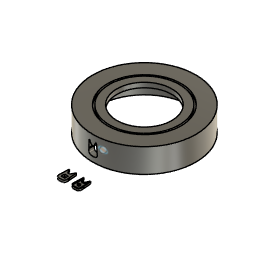
PLAtaforma v2 (Autodesk Fusion 360 design; units mm, degrees)
Autodesk Fusion 360 part; units mm, degrees
sketch "Boceto1" plane through (0, 0, 0) normal (0, 0, 1) x (1, 0, 0)
  circle A0 centre (-125, 125) radius 55.5
sketch "Boceto2" plane through (0, 0, 0) normal (0, 0, 1) x (1, 0, 0)
  circle A0 centre (0, 27.0396) radius 57.4187
  circle A1 centre (150, 200) radius 57.5
extrude "Extruir3" add sketch "Boceto2" along normal blind 35 contours A1 makes body 1
move_body "Desplazar4" bodies 1 to x (1, 0, 0) y (0, 1, 0) z (0, 0, 1) at (-150, -175, 50)
sketch "Boceto3" plane through (0, 0, 85) normal (0, 0, 1) x (-1, 0, 0)
  circle A0 centre (0, -25) radius 57.5
  circle A1 centre (0, -25) radius 40
  constraint concentric A0 A1
extrude "Extruir4" cut sketch "Boceto3" against normal blind 40 contours A1 bodies 1
sketch "Boceto4" plane through (0, 0, 85) normal (0, 0, 1) x (-1, 0, 0)
  circle A0 centre (0, -25) radius 40
  circle A1 centre (0, -25) radius 57.5
move_body "Desplazar5" bodies 1 to x (1, 0, 0) y (0, 1, 0) z (0, 0, 1) at (0, 0, -140)
sketch "Boceto5" plane through (0, 0, -55) normal (0, 0, 1) x (-1, 0, 0)
  circle A0 centre (0, -25) radius 40
  circle A1 centre (0, -25) radius 57.5
  circle A2 centre (0, -25) radius 53.4509
  circle A3 centre (0, -25) radius 51
  constraint concentric A0 A2
  constraint concentric A0 A3
extrude "Extruir5" cut sketch "Boceto5" against normal blind 3 contours A2 bodies 1
fillet "Empalme1" radius 0.25 1 edges at (49.8337, 5.6713, -58) on bodies 1
fillet "Empalme2" radius 0.25 1 edges at (47.5487, 43.4424, -58) on bodies 1
sketch "Boceto6" plane through (0, 0, -55) normal (0, 0, 1) x (-1, 0, 0)
  circle A0 centre (0, -25) radius 51
  circle A1 centre (0, -25) radius 40
  line L0 (100, -175) -> (45.9317, -175)
  line L1 (45.9317, -175) -> (45.9317, -137.795)
  line L2 (45.9317, -137.795) -> (100, -137.795)
  line L3 (100, -137.795) -> (100, -175)
  constraint horizontal L0
  constraint vertical L1
  constraint horizontal L2
  constraint vertical L3
sketch "Boceto7" plane through (0, 0, 0) normal (0, 1, 0) x (1, 0, 0)
  spline S0 degree 5 poles (-6, -14) (-6.016, -13.81) (-6.046, -13.4349) (-6.0844, -12.8873) (-6.1226, -12.187) (-6.143, -11.3625) (-6.116, -10.5901) (-6.0091, -9.873) (-5.7505, -9.2135) (-5.2931, -8.6238) (-4.6335, -8.1243) (-3.7909, -7.7338) (-2.8029, -7.4645) (-1.7133, -7.3125) (-0.5683, -7.2594) (0.5856, -7.2827) (1.7041, -7.3621) (2.7474, -7.489) (3.6824, -7.6725) (4.4854, -7.9512) (5.1429, -8.3847) (5.6471, -9.0113) (5.9972, -9.8345) (6.1897, -10.7563) (6.235, -11.6318) (6.1815, -12.4467) (6.1039, -13.0649) (6.0484, -13.5294) (6.0154, -13.8425) (6, -14) knots 0 0 0 0 0 0 0.04 0.08 0.12 0.16 0.2 0.24 0.28 0.32 0.36 0.4 0.44 0.48 0.52 0.56 0.6 0.64 0.68 0.72 0.76 0.8 0.84 0.88 0.92 0.96 1 1 1 1 1 1
  line L0 (6.1425, -12.5468) -> (5.8575, -15.4532)
  line L1 (5.5566, -8.4249) -> (6.4434, -11.5751)
  line L2 (-6.2996, -11.2694) -> (-5.7004, -8.7306)
  spline S1 degree 5 poles (-5.8636, -15.4223) (-5.8656, -16.3931) (-5.8678, -18.2327) (-5.8657, -20.6855) (-5.8432, -23.3299) (-5.7393, -25.5443) (-5.5105, -26.6441) (-5.1266, -26.6944) (-4.5821, -25.8579) (-3.9459, -24.5382) (-3.2994, -23.1771) (-2.6763, -22.0178) (-2.1679, -21.2779) (-1.777, -20.8414) (-1.5201, -20.6109) (-1.4081, -20.5209) knots 0 0 0 0 0 0 0.04 0.08 0.12 0.16 0.2 0.24 0.28 0.32 0.36 0.4 0.430271 0.430271 0.430271 0.430271 0.430271 0.430271
  line L3 (-5.8558, -11.6968) -> (-5.8714, -19.1478)
  line L4 (-4.7611, -26.105) -> (-4.2835, -25.2366)
  ellipse E0 centre (0, -14) end of major axis (6, -14) minor radius 6.7082 (-6, -14) -> (-5.8636, -15.4223) ccw
  ellipse E1 centre (0, -14) end of major axis (6, -14) minor radius 6.7082 (-1.4081, -20.5209) -> (1.0288, -20.6089) ccw
  ellipse E2 centre (0, -14) end of major axis (6, -14) minor radius 6.7082 (5.8575, -15.4532) -> (6, -14) ccw
  spline S2 degree 5 poles (1.0288, -20.6089) (1.0454, -20.6251) (1.2133, -20.7918) (1.5263, -21.1625) (1.9673, -21.8512) (2.5023, -22.9747) (3.0752, -24.4534) (3.5768, -25.7819) (4.0187, -26.6987) (4.4124, -26.9878) (4.766, -26.5076) (5.0852, -25.1698) (5.3736, -22.9285) (5.5812, -20.3988) (5.7243, -18.0869) (5.814, -16.3617) (5.8575, -15.4532) knots 0.555614 0.555614 0.555614 0.555614 0.555614 0.555614 0.56 0.6 0.64 0.68 0.72 0.76 0.8 0.84 0.88 0.92 0.96 1 1 1 1 1 1
  line L5 (0.2621, -19.8617) -> (1.7954, -21.356)
  line L6 (5.6884, -18.9867) -> (6.0267, -11.9197)
  spline S3 degree 3 poles (-1.4604, -20.264) (-0.626, -20.5082) (0.2565, -20.5396) (1.1028, -20.3557) knots 2.884408 2.884408 2.884408 2.884408 3.334897 3.334897 3.334897 3.334897
  spline S4 degree 3 poles (1.1028, -20.3557) (1.1323, -20.3844) (1.1619, -20.4132) (1.1914, -20.442) (1.9144, -21.1466) (2.5155, -22.4275) (3.0242, -23.696) (3.3295, -24.4573) (3.6018, -25.1998) (3.8432, -25.7413) (4.0212, -26.1408) (4.1959, -26.4325) (4.2994, -26.53) (4.3198, -26.5492) (4.3362, -26.5607) (4.346, -26.5662) knots 0.550938 0.550938 0.550938 0.550938 0.555614 0.555614 0.555614 0.661996 0.661996 0.661996 0.725847 0.725847 0.725847 0.772953 0.772953 0.772953 0.78222 0.78222 0.78222 0.78222
  spline S5 degree 3 poles (4.346, -26.5662) (4.3827, -26.5368) (4.4823, -26.3889) (4.5725, -26.1162) (4.9775, -24.8912) (5.343, -21.3299) (5.6248, -15.4421) (5.6251, -15.4363) (5.6253, -15.4305) (5.6256, -15.4247) knots 0.80969 0.80969 0.80969 0.80969 0.844339 0.844339 0.844339 1 1 1 1.000153 1.000153 1.000153 1.000153
  spline S6 degree 3 poles (5.6256, -15.4247) (5.7202, -14.954) (5.7677, -14.4713) (5.767, -13.9887) knots -1.791812 -1.791812 -1.791812 -1.791812 -1.569057 -1.569057 -1.569057 -1.569057
  spline S7 degree 3 poles (-5.767, -13.9903) (-5.7673, -13.987) (-5.7676, -13.9837) (-5.7678, -13.9804) (-5.8747, -12.715) (-5.9561, -11.5732) (-5.8629, -10.6164) (-5.7828, -9.7954) (-5.5171, -9.1267) (-4.8246, -8.5921) (-4.0701, -8.0096) (-2.8284, -7.6532) (-1.4477, -7.5498) (-0.0784, -7.4473) (1.4043, -7.5365) (2.616, -7.7229) (3.7061, -7.8906) (4.542, -8.1517) (5.0887, -8.7456) (5.479, -9.1697) (5.7466, -9.8087) (5.8761, -10.4922) (6.0308, -11.3093) (5.9793, -12.0858) (5.8969, -12.8241) (5.8544, -13.2054) (5.8064, -13.5869) (5.7681, -13.9773) (5.7677, -13.9811) (5.7674, -13.9849) (5.767, -13.9887) knots -0.000415 -0.000415 -0.000415 -0.000415 0 0 0 0.160546 0.160546 0.160546 0.298298 0.298298 0.298298 0.448379 0.448379 0.448379 0.597213 0.597213 0.597213 0.731122 0.731122 0.731122 0.82672 0.82672 0.82672 0.940992 0.940992 0.940992 1 1 1 1.000581 1.000581 1.000581 1.000581
  spline S8 degree 3 poles (-5.767, -13.9903) (-5.7676, -14.4639) (-5.7217, -14.9376) (-5.6305, -15.4) knots 1.569298 1.569298 1.569298 1.569298 1.787916 1.787916 1.787916 1.787916
  spline S9 degree 3 poles (-5.6305, -15.4) (-5.6306, -15.4076) (-5.6306, -15.4152) (-5.6306, -15.4228) (-5.6379, -18.9007) (-5.6384, -21.5996) (-5.58, -23.4507) (-5.5465, -24.5102) (-5.4905, -25.2917) (-5.4051, -25.7776) (-5.3556, -26.0591) (-5.2879, -26.2439) (-5.248, -26.3044) knots -0.000188 -0.000188 -0.000188 -0.000188 0 0 0 0.085991 0.085991 0.085991 0.13521 0.13521 0.13521 0.163732 0.163732 0.163732 0.163732
  spline S10 degree 3 poles (-5.248, -26.3044) (-5.1951, -26.267) (-5.0881, -26.1485) (-4.9745, -25.9761) (-4.6357, -25.4621) (-4.1975, -24.5076) (-3.7667, -23.6307) (-3.1866, -22.4499) (-2.5988, -21.3794) (-1.925, -20.6804) (-1.8044, -20.5553) (-1.6809, -20.4412) (-1.554, -20.3392) (-1.5228, -20.3142) (-1.4916, -20.2891) (-1.4604, -20.264) knots 0.197683 0.197683 0.197683 0.197683 0.224372 0.224372 0.224372 0.303955 0.303955 0.303955 0.411102 0.411102 0.411102 0.430271 0.430271 0.430271 0.435327 0.435327 0.435327 0.435327
  spline S11 degree 3 poles (-1.6069, -19.4391) (-0.6663, -19.7925) (0.3605, -19.8343) (1.3181, -19.5394) knots 2.809731 2.809731 2.809731 2.809731 3.412393 3.412393 3.412393 3.412393
  spline S12 degree 3 poles (1.3181, -19.5394) (1.4468, -19.6649) (1.5756, -19.7903) (1.7043, -19.9157) (2.5333, -20.7237) (3.1086, -21.9593) (3.6075, -23.1786) (3.8069, -23.6658) (3.9901, -24.1463) (4.1575, -24.5734) knots 0.535231 0.535231 0.535231 0.535231 0.555614 0.555614 0.555614 0.655325 0.655325 0.655325 0.695165 0.695165 0.695165 0.695165
  spline S13 degree 3 poles (4.1575, -24.5734) (4.3953, -23.0694) (4.6167, -20.5464) (4.8059, -17.071) (4.8349, -16.5389) (4.8632, -15.9842) (4.8908, -15.4069) (4.892, -15.3822) (4.8932, -15.3574) (4.8944, -15.3327) knots 0.884759 0.884759 0.884759 0.884759 0.984699 0.984699 0.984699 1 1 1 1.000654 1.000654 1.000654 1.000654
  spline S14 degree 3 poles (4.8944, -15.3327) (4.9887, -14.8822) (5.0352, -14.418) (5.032, -13.9543) knots -1.801106 -1.801106 -1.801106 -1.801106 -1.562974 -1.562974 -1.562974 -1.562974
  spline S15 degree 3 poles (-5.0321, -13.9606) (-5.0332, -13.9466) (-5.0344, -13.9326) (-5.0356, -13.9186) (-5.1324, -12.7725) (-5.1982, -11.718) (-5.148, -10.8988) (-5.114, -10.343) (-5.0256, -9.9608) (-4.8186, -9.6427) (-4.5793, -9.2749) (-4.111, -8.9111) (-3.3636, -8.6522) (-2.1935, -8.2468) (-0.4069, -8.1825) (1.1858, -8.3027) (2.3016, -8.3869) (3.3078, -8.5464) (3.9025, -8.8031) (4.3809, -9.0095) (4.6377, -9.2478) (4.8704, -9.7298) (5.1052, -10.2159) (5.235, -10.9178) (5.2421, -11.548) (5.2507, -12.3058) (5.1191, -13.0657) (5.0368, -13.9056) (5.0352, -13.9218) (5.0336, -13.9381) (5.032, -13.9543) knots -0.00177 -0.00177 -0.00177 -0.00177 0 0 0 0.147475 0.147475 0.147475 0.247541 0.247541 0.247541 0.363232 0.363232 0.363232 0.544362 0.544362 0.544362 0.671249 0.671249 0.671249 0.7733 0.7733 0.7733 0.876232 0.876232 0.876232 1 1 1 1.002476 1.002476 1.002476 1.002476
  spline S16 degree 3 poles (-5.0321, -13.9606) (-5.0348, -14.4203) (-4.9886, -14.8803) (-4.8956, -15.3269) knots 1.564057 1.564057 1.564057 1.564057 1.800092 1.800092 1.800092 1.800092
  spline S17 degree 3 poles (-4.8956, -15.3269) (-4.8956, -15.3594) (-4.8957, -15.3919) (-4.8958, -15.4243) (-4.9024, -18.5904) (-4.9025, -21.1111) (-4.8595, -22.9176) (-4.849, -23.3605) (-4.8356, -23.7598) (-4.8188, -24.1144) knots -0.000803 -0.000803 -0.000803 -0.000803 0 0 0 0.07832 0.07832 0.07832 0.09752 0.09752 0.09752 0.09752
  spline S18 degree 3 poles (-4.8188, -24.1144) (-4.6256, -23.7164) (-4.4261, -23.3008) (-4.2221, -22.8962) (-3.5866, -21.6364) (-2.9314, -20.5033) (-2.0143, -19.7664) (-1.8785, -19.6573) (-1.7427, -19.5482) (-1.6069, -19.4391) knots 0.279655 0.279655 0.279655 0.279655 0.31626 0.31626 0.31626 0.430271 0.430271 0.430271 0.452279 0.452279 0.452279 0.452279
  point P0 (-6, -10)
  point P1 (-3.3594, -7.636)
  point P2 (3.1902, -7.5882)
  point P3 (6, -10)
  point P4 (3.8918, -26.3618)
  dimension "d24" = 0.233
  dimension "d27" = -0.9678
  constraint midpoint S0.end L0
  constraint midpoint P3 L1
  constraint midpoint P0 L2
  constraint coincident S2.start E0
  constraint coincident L0.end S2.end
  constraint midpoint S1.start L3
  constraint coincident S1 S1.end
  constraint concentric E0 E1
  constraint concentric E1 E2
  constraint midpoint S2.start L5
  constraint midpoint L0.end L6
move_body "Desplazar6" bodies 1 to x (1, 0, 0) y (0, 1, 0) z (0, 0, 1) at (0, 0, 90)
move_body "Desplazar7" bodies 1 to x (1, 0, 0) y (0, 1, 0) z (0, 0, 1) at (0, 35, 0)
extrude "Extruir7" cut sketch "Boceto7" along normal blind 28 contours S0 L0 L3 E0 S2 L5 S3 S4 S5 S6 S7 | S1 L3 E1 L5 S3 S7 S8 S9 S10 | S3 S4 S5 S6 S7 S8 S9 S10 | L0 E2 | S11 S12 S13 S14 S15 S16 S17 S18 bodies 1
extrude "Extruir8" add sketch "Boceto7" along normal blind 3 separate body contours S3 S4 S5 S6 S7 S8 S9 S10 | S11 S12 S13 S14 S15 S16 S17 S18 makes body 2
extrude "Extruir9" cut sketch "Boceto7" along normal blind 1 contours S11 S12 S13 S14 S15 S16 S17 S18 bodies 2
move_body "Desplazar8" bodies 2 to x (1, 0, 0) y (0, 1, 0) z (0, 0, 1) at (0, 2, 0)
move_body "Desplazar9" bodies 2 to x (1, 0, 0) y (0, 1, 0) z (0, 0, 1) at (0, -15, 0)
sketch "Boceto8" plane through (0, 0, 0) normal (0, 1, 0) x (1, 0, 0)
  circle A0 centre (0, -14) radius 1.5
  circle A1 centre (0, -14) radius 1.8943
  dimension "d30" = 3
  dimension "d31" = 0.3943
  measures "d30" diameter of A0
extrude "Extruir10" add sketch "Boceto8" against normal blind 1 separate body makes body 3
move_body "Desplazar10" bodies 3 to x (1, 0, 0) y (0, 1, 0) z (0, 0, 1) at (0, -12, 0)
sketch "Boceto9" plane through (0, 0, 0) normal (0, 1, 0) x (1, 0, 0)
  line L0 (-2.5, -16.5) -> (2.6, -16.5)
  line L1 (2.6, -16.5) -> (2.6, -11.4)
  line L2 (2.6, -11.4) -> (-2.5, -11.4)
  line L3 (-2.5, -11.4) -> (-2.5, -16.5)
  dimension "d36" = 5.1
  dimension "d37" = 5.1
  constraint horizontal L0
  constraint vertical L1
  constraint horizontal L2
  constraint vertical L3
  measures "d36" distance of L0.start L0.end
  measures "d37" distance of L0.start L2.end
extrude "Extruir13" add sketch "Boceto7" against normal blind 3 separate body contours S3 S4 S5 S6 S7 S8 S9 S10 | S11 S12 S13 S14 S15 S16 S17 S18 makes body 4
extrude "Extruir14" cut sketch "Boceto9" against normal blind 5 bodies 4
sketch "Boceto10" plane through (0, 0, 0) normal (0, 0, 1) x (1, 0, 0)
hole "Agujero2" at (-30.1866, 23.4332, 0) direction (0, 0, 1) diameter 1.623 depth 15 tip angle 118 countersink diameter 6 countersink angle 90 bodies 1
thread "Rosca2" "ISO Metric profile 2.0 M2x0.4 M2x0.4 6H" thread offset 0 thread depth 7.4
hole "Agujero3" at (30.5773, 23.6208, 0) direction (0, 0, 1) diameter 1.623 depth 15 tip angle 118 countersink diameter 6 countersink angle 90 bodies 1
thread "Rosca3" "ISO Metric profile 2.0 M2x0.4 M2x0.4 6H" thread offset 0 thread depth 7.4
hole "Agujero4" at (-30.0936, 95.2309, 0) direction (0, 0, 1) diameter 1.623 depth 15 tip angle 118 countersink diameter 6 countersink angle 90 bodies 1
thread "Rosca4" "ISO Metric profile 2.0 M2x0.4 M2x0.4 6H" thread offset 0 thread depth 7.4
hole "Agujero5" at (31.1473, 95.0805, 0) direction (0, 0, 1) diameter 1.623 depth 15 tip angle 118 countersink diameter 6 countersink angle 90 bodies 1
thread "Rosca5" "ISO Metric profile 2.0 M2x0.4 M2x0.4 6H" thread offset 0 thread depth 7.4
sketch "Boceto11" plane through (0, 0, 0) normal (0, 0, 1) x (1, 0, 0)
  circle A0 centre (0, 60) radius 42.5957
move_body "Desplazar11" bodies 1 to x (1, 0, 0) y (0, 1, 0) z (0, 0, 1) at (0, 0, -5)
extrude "Extruir15" cut sketch "Boceto11" along normal blind 25 bodies 1
sketch "Boceto12" plane through (0, 0, 0) normal (0, 1, 0) x (1, 0, 0)
sketch "Boceto13" plane through (0, 0, 0) normal (0, 1, 0) x (1, 0, 0)
sketch "Boceto14" plane through (0, 0, 0) normal (0, 1, 0) x (1, 0, 0)
  circle A0 centre (-0.0804, -7.7307) radius 3
  dimension "d75" = 6
  measures "d75" diameter of A0
extrude "Extruir16" cut sketch "Boceto14" along normal blind 125 bodies 1
move_body "Desplazar12" bodies 3 to x (1, 0, 0) y (0, 1, 0) z (0, 0, 1) at (0, -5, 0)
sketch "Boceto15" plane through (0, 0, -5) normal (0, 0, -1) x (1, 0, 0)
  circle A0 centre (31.1473, -95.0805) radius 3
  circle A1 centre (-30.0936, -95.2309) radius 3
  circle A2 centre (30.5773, -23.6208) radius 3
  circle A3 centre (-30.1866, -23.4332) radius 3
  circle A4 centre (0, -60) radius 40
  circle A5 centre (0, -60) radius 57.5
  circle A6 centre (-30.1866, -23.4332) radius 5.3169
  circle A7 centre (30.5773, -23.6208) radius 4.9243
  circle A8 centre (31.1473, -95.0805) radius 5.6219
  circle A9 centre (-30.0936, -95.2309) radius 4.6387
  constraint concentric A3 A6
  constraint concentric A2 A7
  constraint concentric A0 A8
  constraint concentric A1 A9
extrude "Extruir17" add sketch "Boceto15" against normal blind 20 contours A0 | A1 | A2 | A3 | A6 | A7 | A8 | A9 bodies 1
move_body "Desplazar13" bodies 3 to x (1, 0, 0) y (0, 1, 0) z (0, 0, 1) at (0, 5, 0)
delete_face "SuprimirCaras1" 1 faces at (-25.9876, 93.0725, 5) on bodies 1
delete_face "SuprimirCaras2" 1 faces at (-26.9925, 27.6837, 10) on bodies 1
hole "Agujero6" at (36.6643, 27.8536, -5) direction (0, 0, 1) diameter 2 depth 20 tip angle 118 bodies 1
hole "Agujero7" at (35.4013, 92.2882, -5) direction (0, 0, 1) diameter 2 depth 20 tip angle 118 bodies 1
hole "Agujero8" at (-34.8553, 26.4139, -5) direction (0, 0, 1) diameter 2 depth 20 tip angle 118 bodies 1
hole "Agujero9" at (-36.0064, 92.1661, -5) direction (0, 0, 1) diameter 2 depth 20 tip angle 118 bodies 1
sketch "Boceto16" plane through (0, 0, 0) normal (0, 0, 1) x (1, 0, 0)
  circle A0 centre (0, 60) radius 75
  circle A1 centre (0, 60) radius 53.4478
  circle A2 centre (0, 60) radius 51.0031
  circle A3 centre (0, 60) radius 39.9912
  circle A4 centre (0, 60) radius 67.082
  dimension "d92" = 150
  constraint concentric A0 A1
  constraint concentric A0 A2
  constraint concentric A2 A3
  constraint concentric A2 A4
  measures "d92" diameter of A0
extrude "Extruir19" add sketch "Boceto16" along normal blind 35 separate body contours A0 | A2 | A4 makes body 5 at (74.6273, 52.5324, 23.3333) makes body 6 at (50.7496, 54.9217, 23.3333)
extrude "Extruir21" add sketch "Boceto16" along normal blind 32 contours A1 bodies 6
extrude "Extruir22" cut sketch "Boceto16" along normal blind 28 contours A1 | A2 | A4 bodies 5 6
extrude "Extruir23" cut sketch "Boceto7" against normal blind 24 contours S0 L0 L3 E0 S2 L5 S3 S4 S5 S6 S7 | S1 L3 E1 L5 S3 S7 S8 S9 S10 | S3 S4 S5 S6 S7 S8 S9 S10 | L0 E2 | S11 S12 S13 S14 S15 S16 S17 S18 bodies 5
move_body "Desplazar14" bodies 3 2 4 to x (1, 0, 0) y (0, 0, -1) z (0, 1, 0) at (0, -70.1057, -0.8943)
move_body "Desplazar15" bodies 3 2 to x (1, 0, 0) y (0, 1, 0) z (0, 0, 1) at (21, 0, -10)
move_body "Desplazar16" bodies 2 4 3 to x (1, 0, 0) y (0, 1, 0) z (0, 0, 1) at (0, 0, 0.9)
sketch "Boceto17" plane through (0, 0, 0) normal (0, 1, 0) x (1, 0, 0)
  ellipse E0 centre (0, -8) end of major axis (-6, -8) minor radius 3.1723
  line L0 (6, -8) -> (-6, -8) construction
  line L1 (0, -4.8277) -> (0, -11.1723) construction
  dimension "d105" = 12
  constraint coincident E0 L0.start
  constraint coincident E0 L0.end
  constraint coincident E0 L1.start
  constraint coincident E0 L1.end
  constraint horizontal L0
  measures "d105" distance of E0
named bodies: "base", "boton forma", "boton", "hold"
